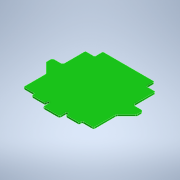
# Autodesk Inventor part: MainBoard
Saved by Autodesk Inventor 2021 (Build 250183000, 183)
## iProperties
Created: 2021-05-13
Part Number: MainBoard
Material: Generic
Document SubType Name: Modeling
Designer: ermoz
Density: 1 g/cm^3
Appearance: Default
Author: ermoz
Autodesk Inventor part; units mm, degrees
ref_plane "YZ Plane" through (0, 0, 0) normal (1, 0, 0) x (0, 1, 0)
ref_plane "XZ Plane" through (0, 0, 0) normal (0, 1, 0) x (-1, 0, 0)
ref_plane "XY Plane" through (0, 0, 0) normal (0, 0, 1) x (1, 0, 0)
sketch "Sketch1" plane through (0, 0, 0) normal (0, 1, 0) x (-1, 0, 0)
  line L0 (-25, -37.5) -> (25, -37.5)
  line L1 (25, -37.5) -> (25, 30.5)
  line L2 (25, 30.5) -> (-25, 30.5)
  line L3 (-25, 30.5) -> (-25, -37.5)
  line L4 (-25, -37.5) -> (25, 30.5) construction
  line L5 (25, -37.5) -> (-25, 30.5) construction
  point P0 (0, -3.5)
  point P1 (0, -3.5)
  point P2 (0, -3.5)
  dimension "d0" = 68
  dimension "d1" = 50
  constraints: 12 end point, 4 midpoint, 2 horizontal, 2 parallel, 1 perpendicular
  measures "d0" distance of L0.end L1.end
  measures "d1" distance of L1.end L2.end
extrude "Extrusion1" add sketch "Sketch1" along normal blind 1.6
sketch "Sketch2" plane through (0, 0, 0) normal (0, -1, 0) x (1, 0, 0)
  line L0 (25, 30.5) -> (25, -37.5) projected
  line L1 (25, -29.5) -> (34, -29.5)
  line L2 (34, -29.5) -> (34, 30.5)
  line L3 (34, 30.5) -> (25, 30.5)
  line L4 (25, 30.5) -> (25, -29.5)
  line L5 (-25, -37.5) -> (-25, 30.5) projected
  line L6 (-25, -29.5) -> (-34, -29.5)
  line L7 (-34, -29.5) -> (-34, 30.5)
  line L8 (-34, 30.5) -> (-25, 30.5)
  line L9 (-25, 30.5) -> (-25, -29.5)
  line L10 (25, -37.5) -> (-25, -37.5) projected
  line L11 (-8, 37.5) -> (8, 37.5)
  line L12 (8, 37.5) -> (8, 30.5)
  line L13 (8, 30.5) -> (-8, 30.5)
  line L14 (-8, 30.5) -> (-8, 37.5)
  line L15 (-8, 37.5) -> (8, 30.5) construction
  line L16 (8, 37.5) -> (-8, 30.5) construction
  line L17 (-25, 30.5) -> (25, 30.5) projected
  line L18 (25, 30.5) -> (10, 30.5)
  line L19 (10, 30.5) -> (10, 33.5)
  line L20 (10, 33.5) -> (23, 33.5)
  line L21 (23, 33.5) -> (23, 30.5)
  line L22 (-25, 30.5) -> (-10, 30.5)
  line L23 (-10, 30.5) -> (-10, 33.5)
  line L24 (-10, 33.5) -> (-23, 33.5)
  line L25 (-23, 33.5) -> (-23, 30.5)
  point P0 (0, 0)
  point P1 (25, 28.5)
  point P2 (25, -35.5)
  point P3 (-25, -35.5)
  point P4 (-25, 28.5)
  point P5 (23, 30.5)
  point P6 (23, -37.5)
  point P7 (-23, -37.5)
  point P8 (25, 23.5)
  point P9 (-25, 23.5)
  point P10 (25, 28.5)
  point P11 (-25, 28.5)
  point P12 (0, 34)
  point P13 (0, 34)
  point P14 (0, 30.5)
  point P15 (10, 30.5)
  point P16 (23, 30.5)
  dimension "d5" = 9
  dimension "d6" = 9
  dimension "d8" = 8
  dimension "d12" = 16
  dimension "d13" = 7
  dimension "d14" = 3
  dimension "d15" = 13
  dimension "d16" = 2
  dimension "d17" = 2
  constraints: 44 end point, 10 parallel, 5 horizontal, 5 perpendicular, 5 point on line, 4 midpoint, 2 collinear, 1 vertical alignment
  measures "d5" distance of L0.start L2.end
  measures "d6" distance of L7.end L5.end
  measures "d8" distance between parallel lines of L10 L6
  measures "d12" distance of L12.end L13.end
  measures "d13" distance of L11.end L12.end
  measures "d14" distance between parallel lines of L17 L20
  measures "d15" distance of L19.end L20.end
  measures "d16" distance between parallel lines of L0 L21
  measures "d17" distance between parallel lines of L9 L25
extrude "Extrusion2" add sketch "Sketch2" against normal up to surface (1.6 mm away) contours L3 L2 L1 L0 | L17 L19 L20 L21 | L13 L14 L11 L12 | L6 L7 L8 L5 | L17 L25 L24 L23
fillet "Fillet2" radius 1 20 edges at (-34, 0.8, 30.5) (-25, 0.8, -29.5) (-34, 0.8, -29.5) (25, 0.8, -29.5) (34, 0.8, -29.5) (34, 0.8, 30.5) (25, 0.8, -37.5) (-25, 0.8, -37.5) (8, 0.8, 30.5) (8, 0.8, 37.5) (-8, 0.8, 37.5) (-8, 0.8, 30.5) (23, 0.8, 33.5) (10, 0.8, 33.5) (10, 0.8, 30.5) (-10, 0.8, 30.5) (-10, 0.8, 33.5) (-23, 0.8, 33.5) (-23, 0.8, 30.5) (23, 0.8, 30.5)
sketch "Sketch3" plane through (0, 1.6, 0) normal (0, 1, 0) x (1, 0, 0)
  line L0 (34, 28.5) -> (34, -29.5) projected
  line L1 (34, -8.5) -> (44, -8.5)
  line L2 (44, -8.5) -> (44, 7.5)
  line L3 (44, 7.5) -> (34, 7.5)
  line L4 (34, 7.5) -> (34, -8.5)
  line L5 (-34, -29.5) -> (-34, 28.5) projected
  line L6 (-34, -8.5) -> (-44, -8.5)
  line L7 (-44, -8.5) -> (-44, 7.5)
  line L8 (-44, 7.5) -> (-34, 7.5)
  line L9 (-34, 7.5) -> (-34, -8.5)
  line L10 (24, -30.5) -> (33, -30.5) projected
  point P0 (0, 0)
  point P1 (34, 7.5)
  dimension "d18" = 10
  dimension "d19" = 16
  dimension "d20" = 10
  dimension "d21" = 22
  constraints: 16 end point, 4 parallel, 4 point on line, 2 horizontal, 2 perpendicular
  measures "d18" distance of L3.end L2.end
  measures "d19" distance of L2.end L1.end
  measures "d20" distance of L7.end L8.end
  measures "d21" distance between parallel lines of L10 L1
extrude "Extrusion3" add sketch "Sketch3" against normal up to surface (1.6 mm away)
sketch "Sketch4" plane through (0, 1.6, 0) normal (0, 1, 0) x (1, 0, 0)
  line L0 (-44, -8.5) -> (-34, -8.5) projected
  line L1 (-34, -8.5) -> (-44, 1.5)
  line L2 (-44, -8.5) -> (-44, 7.5) projected
  line L3 (-34, -8.5) -> (-19.8579, -8.5) construction
  line L4 (44, -8.5) -> (34, -8.5) projected
  line L5 (34, -8.5) -> (44, 1.5)
  line L6 (44, 7.5) -> (44, -8.5) projected
  line L7 (34, -8.5) -> (48.1421, -8.5) construction
  line L8 (-44, 1.5) -> (-44, -8.5)
  line L9 (-44, -8.5) -> (-34, -8.5)
  line L10 (34, -8.5) -> (44, -8.5)
  line L11 (44, -8.5) -> (44, 1.5)
  point P0 (0, 0)
  dimension "d24" = 135
  dimension "d25" = 45
  dimension "d26" = 10
  dimension "d27" = 10
  constraints: 16 end point, 4 point on line, 2 collinear, 2 equal length, 2 horizontal
  measures "d24" angle of L3 L1
  measures "d25" angle of L7 L5
  measures "d26" distance from line of L2 L1.start
  measures "d27" distance from line of L6 L5.start
extrude "Extrusion4" cut sketch "Sketch4" against normal through all
fillet "Fillet3" radius 2 8 edges at (34, 0.8, 8.5) (44, 0.8, -1.5) (44, 0.8, -7.5) (34, 0.8, -7.5) (-34, 0.8, 8.5) (-44, 0.8, -1.5) (-44, 0.8, -7.5) (-34, 0.8, -7.5)
equation "\"d17\" = d16"
body "Solid1"
